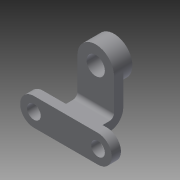
# Autodesk Inventor part: HW 5 Part 6
Saved by Autodesk Inventor 2015 (Build 190159000, 159)
## iProperties
Created: 2016-02-08
Part Number: HW 5 Part 6
Material: Generic
Document SubType Name: Modeling
Designer: Melissa
Density: 1 g/cm^3
Appearance: Default
Author: Melissa
Autodesk Inventor part; units mm, degrees
ref_plane "YZ Plane" through (0, 0, 0) normal (1, 0, 0) x (0, 1, 0)
ref_plane "XZ Plane" through (0, 0, 0) normal (0, 1, 0) x (-1, 0, 0)
ref_plane "XY Plane" through (0, 0, 0) normal (0, 0, 1) x (1, 0, 0)
sketch "Sketch1" plane through (0, 0, 0) normal (0, 0, 1) x (1, 0, 0)
  circle A0 centre (0, 0) radius 25.4
  circle A1 centre (0, 0) radius 50.8
  dimension "d0" = 50.8
  dimension "d1" = 101.6
  constraints: 2 centre point, 2 coincident
  measures "d0" diameter of A0
  measures "d1" diameter of A1
extrude "Extrusion1" add sketch "Sketch1" against normal blind 50.8
sketch "Sketch2" plane through (0, 0, 0) normal (0, 0, 1) x (1, 0, 0)
  circle A0 centre (0, 0) radius 50.8 projected
  line L0 (50.8, 0) -> (50.8, -127)
  line L1 (-50.8, 0) -> (-50.8, -127)
  line L2 (-50.8, -127) -> (50.8, -127)
  circle A1 centre (0, 0) radius 50.8
  dimension "d4" = 127
  dimension "d5" = 127
  dimension "d6" = 101.6
  constraints: 6 end point, 2 point on circle, 2 tangent, 2 vertical, 1 centre point, 1 coincident
  measures "d4" distance of L0.start L0.end
  measures "d5" distance of L1.start L1.end
  measures "d6" diameter of A1
extrude "Extrusion2" add sketch "Sketch2" against normal blind 25.4 contours L0 L2 L1 A0
sketch "Sketch3" plane through (50.8, -127, 0) normal (1, 0, 0) x (0, 0, -1)
  line L0 (0, 0) -> (-57.15, 0)
  line L1 (-57.15, 0) -> (-57.15, 25.4)
  line L2 (-57.15, 25.4) -> (0, 25.4)
  line L3 (0, 25.4) -> (0, 0)
  point P0 (0, 127)
  dimension "d9" = 57.15
  dimension "d10" = 25.4
  constraints: 8 end point, 3 perpendicular, 1 horizontal
  measures "d9" distance of L0.start L0.end
  measures "d10" distance of L0.end L1.end
extrude "Extrusion3" add sketch "Sketch3" against normal blind 101.6
fillet "Fillet1" radius 12.7 1 edges at (0, -101.6, 0)
fillet "Fillet2" radius 38.1 1 edges at (0, -127, -25.4)
sketch "Sketch4" plane through (50.8, -127, 57.15) normal (0, 0, 1) x (1, 0, 0)
  line L0 (-139.7001, 50.8) -> (38.0999, 50.8)
  line L1 (-139.7001, -25.4) -> (38.1001, -25.4)
  arc A0 (-139.7001, 50.8) -> (-139.7001, -25.4) centre (-139.7001, 12.7) ccw
  arc A1 (38.1001, -25.4) -> (38.0999, 50.8) centre (38.1, 12.7) ccw
  line L2 (0, 0) -> (-101.6, 0) projected
  line L3 (-50.8, 0) -> (-50.8, -12.1544)
  line L4 (-50.8, -25.4) -> (-50.8, -31.0464)
  circle A2 centre (-139.7001, 12.7) radius 19.05
  circle A3 centre (38.1, 12.7) radius 19.05
  point P0 (-50.8, 127)
  dimension "d15" = 177.8
  dimension "d16" = 76.2
  dimension "d17" = 38.1
  dimension "d18" = 38.1
  dimension "d20" = 25.4
  dimension "d21" = 0
  dimension "d22" = 38.1
  dimension "d23" = 38.1
  constraints: 8 end point, 4 centre point, 4 point on circle, 2 coincident, 2 midpoint, 2 vertical, 1 horizontal, 1 parallel
  measures "d15" distance of L0.start L0.end
  measures "d16" distance between parallel lines of L0 L1
  measures "d17" radius of A0
  measures "d18" radius of A1
  measures "d20" distance of L4.start L3.start
  measures "d21" horizontal distance of L4.start L3.start
  measures "d22" diameter of A2
  measures "d23" diameter of A3
extrude "Extrusion4" add sketch "Sketch4" along normal blind 25.4
equation "\"d1\" = 2 * d0"
equation "\"d5\" = d4"
equation "\"d17\" = 0.5 * d16"
equation "\"d18\" = d17"
equation "\"d23\" = d22"
body "Solid1"
